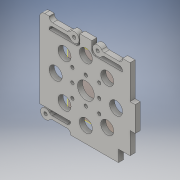
# Autodesk Inventor part: Side
Saved by Autodesk Inventor 2016 (Build 200138000, 138)
## iProperties
Created: 2015-06-30
Part Number: Side
Material: Generic
Document SubType Name: Modeling
Designer: Rodrigo
Density: 1 g/cm^3
Appearance: Default
Author: Rodrigo
Autodesk Inventor part; units mm, degrees
ref_plane "YZ Plane" through (0, 0, 0) normal (1, 0, 0) x (0, 1, 0)
ref_plane "XZ Plane" through (0, 0, 0) normal (0, 1, 0) x (-1, 0, 0)
ref_plane "XY Plane" through (0, 0, 0) normal (0, 0, 1) x (1, 0, 0)
ref_plane "Work Plane1" through (0, 0, 0) normal (0, 0, 1) x (1, 0, 0)
sketch "Sketch1" plane through (0, 0, 0) normal (0, 0, 1) x (1, 0, 0)
  circle A0 centre (6.5, 20.75) radius 1
  circle A1 centre (6.5, 4.75) radius 1
  circle A2 centre (22.5, 20.75) radius 1
  circle A3 centre (22.5, 4.75) radius 1
  line L0 (-13, -14.75) -> (43.896, -14.75)
  line L1 (43.896, -14.75) -> (43.896, 40.25)
  line L2 (43.896, 40.25) -> (-13, 40.25)
  line L3 (-13, 40.25) -> (-13, -14.75)
  circle A4 centre (22.5, 12.75) radius 1 projected
  circle A5 centre (14.5, 20.75) radius 1 projected
  circle A6 centre (14.5, 4.75) radius 1 projected
  circle A7 centre (6.5, 12.75) radius 1 projected
  point P0 (0, 0)
  point P1 (14.5, 12.75)
  dimension "d1" = 55
  dimension "d102" = 29.396
  dimension "d103" = 27.5
  dimension "d107" = 2
  dimension "d108" = 2
  dimension "d109" = 2
  dimension "d110" = 2
  constraints: 8 end point, 4 centre point, 2 parallel, 1 horizontal, 1 perpendicular
  measures "d1" distance of L1.end L0.end
  measures "d102" distance from line of L1 point (14.5, 12.75)
  measures "d103" distance from line of L3 point (14.5, 12.75)
  measures "d107" diameter of A0
  measures "d108" diameter of A2
  measures "d109" diameter of A3
  measures "d110" diameter of A1
extrude "Extrusion3" add sketch "Sketch1" along normal blind 3
sketch "Sketch4" plane through (0, 0, 3) normal (0, 0, 1) x (1, 0, 0)
  line L0 (42, 40.25) -> (-13, 40.25) construction
  line L1 (14.5, 40.25) -> (14.5, 12.75) construction
  line L2 (-13, -14.75) -> (42, -14.75) construction
  line L3 (-13, 40.25) -> (-13, -14.75) construction
  line L4 (-13, 12.75) -> (14.5, 12.75) construction
  circle A0 centre (14.5, 30.75) radius 3.895
  circle A1 centre (1.7721, 25.4779) radius 3.895
  circle A2 centre (-3.5, 12.75) radius 3.895
  circle A3 centre (1.7721, 0.0221) radius 3.895
  circle A4 centre (14.5, -5.25) radius 3.895
  circle A5 centre (27.2279, 0.0221) radius 3.895
  circle A6 centre (32.5, 12.75) radius 3.895
  circle A7 centre (27.2279, 25.4779) radius 3.895
  arc A8 (4.6716, 35.75) -> (4.6716, 37.75) centre (7.5, 36.75) ccw
  line L5 (42, 40.25) -> (-13, 40.25)
  line L6 (7.5, 36.75) -> (-13, 36.75) construction
  line L7 (4.6716, 37.75) -> (-7.3284, 37.75)
  line L8 (4.6716, 35.75) -> (-7.3284, 35.75)
  line L9 (-7.3284, 37.75) -> (-7.3284, 40.25)
  line L10 (10.9716, 40.25) -> (-7.3284, 40.25)
  line L11 (-7.3284, 35.75) -> (-7.3284, 33.25)
  line L12 (-7.3284, 33.25) -> (10.9716, 33.25)
  line L13 (10.9716, 40.25) -> (10.9716, 33.25)
  arc A9 (24.3284, 37.75) -> (24.3284, 35.75) centre (21.5, 36.75) ccw
  line L14 (24.3284, 37.75) -> (36.3284, 37.75)
  line L15 (24.3284, 35.75) -> (36.3284, 35.75)
  line L16 (36.3284, 37.75) -> (36.3284, 40.25)
  line L17 (18.0284, 40.25) -> (36.3284, 40.25)
  line L18 (36.3284, 35.75) -> (36.3284, 33.25)
  line L19 (36.3284, 33.25) -> (18.0284, 33.25)
  line L20 (18.0284, 40.25) -> (18.0284, 33.25)
  arc A10 (-6.6716, -10.25) -> (-6.6716, -12.25) centre (-9.5, -11.25) ccw
  line L21 (-9.5, -11.25) -> (8.4531, -11.25) construction
  line L22 (-6.6716, -10.25) -> (5.3284, -10.25)
  line L23 (-6.6716, -12.25) -> (5.3284, -12.25)
  line L24 (5.3284, -12.25) -> (5.3284, -14.75)
  line L25 (5.3284, -10.25) -> (5.3284, -7.75)
  line L26 (5.3284, -7.75) -> (-13, -7.75)
  line L27 (-13, -14.75) -> (-13, -7.75)
  line L28 (-13, -14.75) -> (5.3284, -14.75)
  circle A11 centre (14.5, 12.75) radius 5
  point P0 (0, 0)
  dimension "d24" = 7.79
  dimension "d25" = 18
  dimension "d28" = 360
  dimension "d63" = 6
  dimension "d64" = 7
  dimension "d65" = 12
  dimension "d66" = 18.3
  dimension "d67" = 2.5
  dimension "d68" = 3.5
  dimension "d71" = 1
  dimension "d74" = 6
  dimension "d75" = 3.5
  dimension "d76" = 3.5
  dimension "d77" = 12
  dimension "d78" = 1
  dimension "d79" = 2.5
  dimension "d105" = 10
  constraints: 58 end point, 14 symmetric about line, 12 centre point, 6 point on circle, 6 point on line, 5 perpendicular, 4 coincident, 4 horizontal, 3 collinear, 3 vertical, 2 midpoint, 18 other
  measures "d24" diameter of A0
  measures "d25" distance of L1.end A0.centre
  measures "d63" diameter of A8
  measures "d64" distance from line of L1 L6.start
  measures "d65" distance of L7.start L7.end
  measures "d66" distance of L10.start L9.end
  measures "d67" distance between parallel lines of L12 L8
  measures "d68" distance from line of L10 L6.start
  measures "d71" distance between parallel lines of L7 L6
  measures "d74" diameter of A10
  measures "d75" distance from line of L21.start L2
  measures "d76" distance from line of L3 L21.start
  measures "d77" distance of L22.start L22.end
  measures "d78" distance between parallel lines of L22 L21
  measures "d79" distance of L22.end L25.end
  measures "d105" diameter of A11
extrude "Extrusion2" cut sketch "Sketch4" against normal through all
hole "Hole4" at (7.5, 36.75, 3) at (21.5, 36.75, 3) at (-9.5, -11.25, 3) direction (0, 0, -1) diameter 2 end through all
fillet "Fillet3" radius 2 14 edges at (-7.3284, 35.75, 1.5) (-7.3284, 37.75, 1.5) (4.6716, 37.75, 1.5) (4.6716, 35.75, 1.5) (10.9716, 33.25, 1.5) (24.3284, 37.75, 1.5) (24.3284, 35.75, 1.5) (36.3284, 37.75, 1.5) (36.3284, 35.75, 1.5) (18.0284, 33.25, 1.5) (5.3284, -10.25, 1.5) (5.3284, -12.25, 1.5) (-6.6716, -10.25, 1.5) (-6.6716, -12.25, 1.5)
sketch "Sketch6" plane through (0, 0, 3) normal (0, 0, 1) x (1, 0, 0)
  line L0 (43.896, 40.25) -> (36.3284, 40.25) projected
  line L1 (43.896, 40.25) -> (40.796, 40.25)
  line L2 (40.796, 40.25) -> (40.796, 20.2)
  line L3 (40.796, 20.2) -> (43.896, 20.2)
  line L4 (43.896, 20.2) -> (43.896, 40.25)
  line L5 (43.896, -14.75) -> (43.896, 40.25) construction
  line L6 (43.896, 12.75) -> (-13, 12.75) construction
  line L7 (-13, 40.25) -> (-13, -7.75) construction
  line L8 (43.896, -14.75) -> (40.796, -14.75)
  line L9 (40.796, -7.75) -> (40.796, 5.3)
  line L10 (40.796, 5.3) -> (43.896, 5.3)
  line L11 (43.896, 5.3) -> (43.896, -14.75)
  line L12 (43.896, -14.75) -> (33.896, -14.75)
  line L13 (33.896, -14.75) -> (33.896, -7.75)
  line L14 (33.896, -7.75) -> (40.796, -7.75)
  line L15 (43.896, -7.75) -> (43.896, -14.75)
  point P0 (0, 0)
  dimension "d96" = 3.1
  dimension "d97" = 20.05
  dimension "d100" = 10
  dimension "d101" = 7
  constraints: 26 end point, 4 parallel, 3 horizontal, 3 symmetric about line, 2 perpendicular, 1 midpoint, 1 point on line
  measures "d96" distance of L3.end L2.end
  measures "d97" distance of L2.end L1.end
  measures "d100" distance of L13.end L15.start
  measures "d101" distance of L12.end L13.end
extrude "Extrusion4" cut sketch "Sketch6" against normal through all
fillet "Fillet4" radius 3 1 edges at (-13, 40.25, 1.5)
equation "\"d38\" = d24"
body "Solid1"
body "Solid2"
